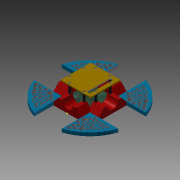
# Autodesk Inventor part: roundBase
Saved by Autodesk Inventor 2015 (Build 190159000, 159)
## iProperties
Created: 2015-10-10
Part Number: roundBase
Material: Generic
Document SubType Name: Modeling
Designer: Ross
Density: 1 g/cm^3
Appearance: Default
Author: Ross
Autodesk Inventor part; units mm, degrees
ref_plane "YZ Plane" through (0, 0, 0) normal (1, 0, 0) x (0, 1, 0)
sketch "Sketch1" plane through (0, 0, 0) normal (0, 1, 0) x (-1, 0, 0)
  line L0 (30.4624, 0) -> (30.4624, 12.4985)
  line L1 (30.4624, 0) -> (30.4624, -12.5)
  line L2 (30.4624, 0) -> (30.4624, 12.4985)
  line L3 (30.4624, 12.4985) -> (37.9972, 12.4985)
  line L4 (30.4624, 12.4985) -> (30.4624, 0)
  line L5 (30.4624, 0) -> (30.4624, -12.5)
  line L6 (30.4624, -12.5) -> (37.9967, -12.5)
  line L7 (-30.5, 0) -> (-30.5, 12.4985)
  line L8 (-30.5, 0) -> (-30.5, -12.4987)
  line L9 (0, 30.5) -> (-12.5, 30.5)
  line L10 (0, 30.5) -> (12.5, 30.5)
  line L11 (0, -30.5) -> (12.5, -30.5)
  line L12 (0, -30.5) -> (-12.5, -30.5)
  line L13 (0, 30.5) -> (12.5, 30.5)
  line L14 (12.5, 30.5) -> (12.5, 37.9967)
  line L15 (0, 30.5) -> (-12.5, 30.5)
  line L16 (-12.5, 30.5) -> (-12.5, 37.9967)
  arc A0 (37.9972, 12.4985) -> (12.5, 37.9967) centre (0, 0) ccw
  arc A1 (12.5, -37.9967) -> (37.9967, -12.5) centre (0, 0) ccw
  arc A2 (-12.5, 37.9967) -> (-37.9972, 12.4985) centre (0, 0) ccw
  arc A3 (-37.9972, -12.4985) -> (-12.5, -37.9967) centre (0, 0) ccw
  line L17 (12.5, -37.9967) -> (12.5, -30.5)
  line L18 (-12.5, -30.5) -> (12.5, -30.5)
  line L19 (-12.5, -30.5) -> (-12.5, -37.9967)
  line L20 (-12.5, -30.5) -> (-12.5, -37.9967)
  line L21 (12.5, -30.5) -> (12.5, -37.9967)
  line L22 (-30.5, 12.4985) -> (-37.9972, 12.4985)
  line L23 (-30.5, -12.4987) -> (-37.9972, -12.4985)
  constraints: 48 end point, 8 point on circle, 6 perpendicular, 4 centre point, 3 vertical, 2 collinear, 1 coincident, 1 point on line
extrude "Extrusion1" add sketch "Sketch1" along normal blind 3
sketch "Sketch4" plane through (30.5, 0, 12.4985) normal (1, 0, 0) x (0, 0, -1)
  line L0 (24.9972, 3) -> (0, 3)
  line L1 (0, 3) -> (0, 0)
  line L2 (0, 0) -> (24.9972, 0)
  line L3 (24.9972, 0) -> (24.9972, 3)
  point P0 (12.4985, 0)
  constraints: 8 end point, 2 parallel, 1 horizontal, 1 perpendicular
extrude "Extrusion4" cut sketch "Sketch4" against normal blind 10
pattern_circular "Circular Pattern2" count 4 over 360 about axis through (0, -10, 0) along (0, 1, 0) of "Extrusion4"
ref_plane "Work Plane1" through (0, 0, 20.5) normal (0, 0, 1) x (1, 0, 0)
sketch "Sketch6" plane through (0, 0, 20.5) normal (0, 0, 1) x (1, 0, 0)
  line L0 (12.4985, 3) -> (-12.4987, 3) projected
  line L1 (-0.0001, 3) -> (4.9999, 3)
  arc A0 (-5.0001, 8) -> (-0.0001, 3) centre (-0.0001, 8) ccw
  arc A1 (-0.0001, 3) -> (4.9999, 8) centre (-0.0001, 8) ccw
  line L2 (-5.0001, 8) -> (-8.0001, 8)
  line L3 (-8.0001, 8) -> (-12.4987, 3)
  line L4 (4.9999, 8) -> (7.9999, 8)
  line L5 (7.9999, 8) -> (12.4985, 3)
  line L6 (-12.4987, 3) -> (12.4985, 3)
  point P0 (0, 0)
  dimension "d30" = 5
  dimension "d32" = 3
  dimension "d33" = 3
  constraints: 12 end point, 4 point on circle, 2 centre point, 1 coincident, 1 collinear, 1 concentric, 1 horizontal, 1 midpoint, 1 parallel, 1 point on line
  measures "d30" distance of L1.start L1.end
  measures "d32" distance of L2.start L2.end
  measures "d33" distance of L4.start L4.end
extrude "Extrusion6" add sketch "Sketch6" against normal blind 10
sketch "Sketch7" plane through (-12.4985, 0, 20.5) normal (0, 0, 1) x (1, 0, 0)
  point P0 (12.4985, 0)
pattern_circular "Circular Pattern3" count 4 over 360 about axis through (0, -10, 0) along (0, 1, 0) of "Extrusion6"
ref_plane "Work Plane2" through (0, 8, 0) normal (0, 1, 0) x (-1, 0, 0)
sketch "Sketch8" plane through (0, 8, 0) normal (0, 1, 0) x (-1, 0, 0)
  circle A0 centre (11.8221, 6.5148) radius 1
  point P0 (0, 0)
  dimension "d40" = 2
  constraints: 1 centre point
  measures "d40" diameter of A0
extrude "Extrusion7" add sketch "Sketch8" along normal blind 7
mirror "Mirror2" about plane through (0, 0, 0) normal (0, 0, 1) of "Extrusion7"
pattern_circular "Circular Pattern4" count 4 over 360 about axis through (0, -10, 0) along (0, 1, 0) of "Extrusion7", "Mirror2"
ref_plane "Work Plane3" through (0, 15, 0) normal (0, 1, 0) x (-1, 0, 0)
sketch "Sketch9" plane through (0, 15, 0) normal (0, 1, 0) x (-1, 0, 0)
  line L0 (-13.8037, -13.7044) -> (13.1963, -13.7044)
  line L1 (13.1963, -13.7044) -> (13.1963, 13.2956)
  line L2 (13.1963, 13.2956) -> (-13.8037, 13.2956)
  line L3 (-13.8037, 13.2956) -> (-13.8037, -13.7044)
  point P0 (0, 0)
  dimension "d47" = 27
  dimension "d48" = 27
  constraints: 8 end point, 2 parallel, 1 horizontal, 1 perpendicular
  measures "d47" distance of L2.end L1.end
  measures "d48" distance of L1.end L0.end
extrude "Extrusion8" add sketch "Sketch9" along normal blind 1
sketch "Sketch10" plane through (0, 16, 0) normal (0, 1, 0) x (1, 0, 0)
  line L0 (7.9999, -20.5) -> (7.9999, -10.5) projected
  line L1 (10.5002, 10.5) -> (7.9999, 10.5)
  line L2 (7.9999, 10.5) -> (7.9999, -10.8221)
  line L3 (7.9999, -10.8221) -> (10.5002, -10.8221)
  line L4 (10.5002, -10.8221) -> (10.5002, 10.5)
  point P0 (0, 0)
  constraints: 8 end point, 2 parallel, 1 horizontal, 1 perpendicular, 1 point on line
extrude "Extrusion9" cut sketch "Sketch10" against normal blind 1
sketch "Sketch15" plane through (0, 3, 0) normal (0, 1, 0) x (1, 0, 0)
  circle A0 centre (-15.0142, 33.7887) radius 1.7857
  point P0 (0, 0)
  constraints: 1 centre point
extrude "Extrusion10" cut sketch "Sketch15" against normal blind 3
pattern_circular "Circular Pattern5" count 4 over 360 about axis through (0, -10, 0) along (0, 1, 0) of "Extrusion10"
sketch "Sketch16" plane through (0, 3, 0) normal (0, 1, 0) x (1, 0, 0)
  circle A0 centre (-14.833, 30.047) radius 1.4657
  circle A1 centre (-17.9901, 31.5127) radius 1.6915
  circle A2 centre (-17.1192, 27.652) radius 1.587
  circle A3 centre (-21.365, 28.9039) radius 2.1773
  circle A4 centre (-14.3431, 25.2025) radius 1.6009
  circle A5 centre (-19.6816, 25.5291) radius 1.252
  circle A6 centre (-17.5517, 24.1107) radius 1.0448
  circle A7 centre (-15.5322, 20.7185) radius 2.3833
  circle A8 centre (-19.1876, 22.6209) radius 0.7565
  circle A9 centre (-21.9753, 25.3714) radius 0.8415
  circle A10 centre (-21.1338, 23.1018) radius 0.9369
  circle A11 centre (-19.0644, 20.4435) radius 1.0376
  circle A12 centre (-17.735, 17.3721) radius 1.4218
  circle A13 centre (-21.1338, 20.8331) radius 0.9881
  circle A14 centre (-20.4855, 17.5555) radius 1.1164
  circle A15 centre (-24.2673, 26.7266) radius 1.0717
  circle A16 centre (-23.0525, 23.8815) radius 0.7028
  circle A17 centre (-25.339, 24.2771) radius 1.4255
  circle A18 centre (-23.7554, 21.3145) radius 1.4848
  circle A19 centre (-22.3497, 18.6719) radius 0.8611
  circle A20 centre (-26.1697, 21.4811) radius 0.7335
  circle A21 centre (-24.2673, 18.3352) radius 0.6743
  circle A22 centre (-19.6816, 14.9197) radius 1.4567
  circle A23 centre (-22.2705, 15.9503) radius 1.1487
  circle A24 centre (-24.7716, 16.0657) radius 1.146
  circle A25 centre (-26.1697, 18.3352) radius 0.7335
  circle A26 centre (-27.3157, 20.1684) radius 0.6895
  circle A27 centre (-28.0053, 23.3774) radius 0.9908
  circle A28 centre (-29.4473, 21.3145) radius 1.0862
  circle A29 centre (-28.0053, 18.5182) radius 0.8803
  circle A30 centre (-27.3157, 16.0657) radius 1.3032
  circle A31 centre (-30.5335, 18.3352) radius 1.3339
  circle A32 centre (-29.4473, 15.3839) radius 0.7207
  circle A33 centre (-31.8674, 16.0657) radius 1.1211
  point P0 (0, 0)
  constraints: 34 centre point
extrude "Extrusion11" cut sketch "Sketch16" against normal blind 3
pattern_circular "Circular Pattern6" count 4 over 360 about axis through (0, -10, 0) along (0, 1, 0) of "Extrusion11"
sketch "Sketch17" plane through (0, 16, 0) normal (0, 1, 0) x (1, 0, 0)
  circle A0 centre (6.5148, 11.8221) radius 1 projected
  circle A1 centre (6.5148, 11.8221) radius 1
  point P0 (0, 0)
  constraints: 1 centre point, 1 coincident
extrude "Extrusion12" cut sketch "Sketch17" against normal blind 1
mirror "Mirror3" about plane through (0, 0, 0) normal (1, 0, 0) of "Extrusion12"
pattern_circular "Circular Pattern7" count 4 over 360 about axis through (0, -10, 0) along (0, 1, 0) of "Extrusion12", "Mirror3"
body "Solid1"
